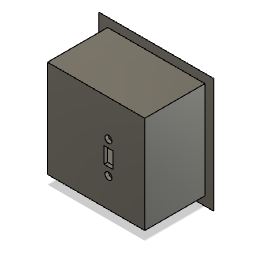
Furniture DC and USB panel v5 (Autodesk Fusion 360 design; units mm, degrees)
Autodesk Fusion 360 part; units mm, degrees
sketch "Sketch1" plane through (0, 0, 0) normal (0, 1, 0) x (1, 0, 0)
  circle A0 centre (0, 0) radius 4.075
  line L0 (26.5, -2.5) -> (17.4, -2.5)
  line L1 (17.4, -2.5) -> (17.4, 2.5)
  line L2 (17.4, 2.5) -> (26.5, 2.5)
  line L3 (26.5, 2.5) -> (26.5, -2.5)
  line L4 (26.5, -2.5) -> (17.4, 2.5) construction
  line L5 (17.4, -2.5) -> (26.5, 2.5) construction
  circle A1 centre (13, 0) radius 2
  circle A2 centre (31, 0) radius 2
  line L6 (-10, 10) -> (41, 10)
  line L7 (41, 10) -> (41, -10)
  line L8 (41, -10) -> (-10, -10)
  line L9 (-10, -10) -> (-10, 10)
  line L10 (-10, 10) -> (-12, 10)
  line L11 (-12, 10) -> (-12, -10)
  line L12 (-12, -10) -> (-10, -10)
  line L13 (-10, -10) -> (-10, 10)
  line L14 (41, 10) -> (43, 10)
  line L15 (43, 10) -> (43, -10)
  line L16 (43, -10) -> (41, -10)
  line L17 (41, -10) -> (41, 10)
  point P0 (21.95, 0)
  dimension "d1" = 8.15
  dimension "d2" = 9.1
  dimension "d3" = 5
  dimension "d4" = 4
  dimension "d5" = 4
  dimension "d6" = 18
  dimension "d7" = 9.05
  dimension "d9" = 13
  dimension "d10" = 10
  dimension "d11" = 10
  dimension "d12" = 10
  dimension "d13" = 10
  dimension "d16" = 51
  constraint coincident A0.centre origin
  constraint perpendicular L0 L1
  constraint parallel L0 L2
  constraint parallel L1 L3
  constraint horizontal L0
  constraint coincident L4 P0
  constraint coincident L5 P0
  constraint horizontal A1.centre A2.centre
  constraint horizontal P0 A2.centre
  constraint horizontal L6
  constraint vertical L7
  constraint horizontal L8
  constraint vertical L9
  constraint horizontal A0.centre A1.centre
  constraint horizontal L10
  constraint vertical L11
  constraint horizontal L12
  constraint vertical L13
  constraint horizontal L14
  constraint vertical L15
  constraint horizontal L16
  constraint vertical L17
  measures "d1" diameter of A0
  measures "d2" distance of L1.end L2.end
  measures "d3" distance of L0.end L1.end
  measures "d4" diameter of A1
  measures "d5" diameter of A2
  measures "d6" distance of A1.centre A2.centre
  measures "d7" horizontal distance of P0 A2.centre
  measures "d9" horizontal distance of A0.centre A1.centre
  measures "d10" distance of A0.centre L9
  measures "d11" distance of A2.centre L7
  measures "d12" distance of A0.centre L8
  measures "d13" distance of A0.centre L6
  measures "d16" distance of L8.end L7.end
extrude "Extrude2" add sketch "Sketch1" along normal blind 2 contours L6 L7 L8 L9 L13 L17 makes body 1
extrude "Extrude1" add sketch "Sketch1" along normal blind 2 separate body contours L6 L7 L8 L9 L13 L17 makes body 2
extrude "Extrude3" add sketch "Sketch1" along normal blind 55 contours L9 L10 L11 L12 L13 | L7 L14 L15 L16 L17 bodies 1 2
sketch "Sketch2" plane through (-10, 0, 0) normal (1, 0, 0) x (0, 0, -1)
  line L0 (-10, 2) -> (10, 2)
  line L1 (10, 2) -> (10, 55)
  line L2 (10, 55) -> (-10, 55)
  line L3 (-10, 55) -> (-10, 2)
  line L4 (-10, 55) -> (10, 55)
  line L5 (10, 55) -> (10, 53)
  line L6 (10, 53) -> (-10, 53)
  line L7 (-10, 53) -> (-10, 55)
  dimension "d21" = 2
  constraint horizontal L4
  constraint vertical L5
  constraint horizontal L6
  constraint vertical L7
  constraint coincident L1 L5.end
  constraint coincident L2.end L3.start
  measures "d21" distance of L4 L6
extrude "Extrude4" add sketch "Sketch2" along normal up to surface (51 mm away) contours L1 L2 L3 L4 L5 L6 L7 bodies 1
sketch "Sketch3" plane through (0, 0, 10) normal (0, 0, 1) x (1, 0, 0)
  line L0 (41, 53) -> (41, 2)
  line L1 (41, 2) -> (-10, 2)
  line L2 (-10, 2) -> (-10, 53)
  line L3 (-10, 53) -> (41, 53)
  line L4 (43, 55) -> (-12, 55)
  line L5 (-12, 55) -> (-12, 0)
  line L6 (-12, 0) -> (43, 0)
  line L7 (43, 0) -> (43, 55)
extrude "Extrude5" add sketch "Sketch3" along normal blind 2 contours L0 L1 L2 L3 | L4 L5 L6 L7 bodies 1
sketch "Sketch4" plane through (0, 0, -10) normal (0, 0, -1) x (-1, 0, 0)
  line L0 (12, 55) -> (-43, 55)
  line L1 (-43, 55) -> (-43, 0)
  line L2 (-43, 0) -> (12, 0)
  line L3 (12, 0) -> (12, 55)
  line L4 (-41, 53) -> (10, 53)
  line L5 (10, 53) -> (10, 2)
  line L6 (10, 2) -> (-41, 2)
  line L7 (-41, 2) -> (-41, 53)
extrude "Extrude6" add sketch "Sketch4" along normal blind 14 bodies 1
sketch "Sketch5" plane through (43, 0, 0) normal (1, 0, 0) x (0, 0, -1)
  line L0 (-12, 0) -> (24, 0)
  line L1 (24, 0) -> (24, 55)
  line L2 (24, 55) -> (-12, 55)
  line L3 (-12, 55) -> (-12, 0)
  line L4 (24, 55) -> (22, 55)
  line L5 (22, 55) -> (22, 0)
  line L6 (22, 0) -> (24, 0)
  line L7 (24, 0) -> (24, 55)
  constraint horizontal L4
  constraint vertical L5
  constraint horizontal L6
  constraint vertical L7
  constraint coincident L0 L5.end
  constraint coincident L1.end L2.start
extrude "Extrude7" add sketch "Sketch5" along normal blind 5 contours L0 L1 L2 L4 L5 L6 L7 bodies 1
sketch "Sketch6" plane through (-12, 0, 0) normal (-1, 0, 0) x (0, 0, 1)
  line L0 (-24, 0) -> (12, 0)
  line L1 (12, 0) -> (12, 55)
  line L2 (12, 55) -> (-24, 55)
  line L3 (-24, 55) -> (-24, 0)
  line L4 (-24, 55) -> (-22, 55)
  line L5 (-22, 55) -> (-22, 0)
  line L6 (-22, 0) -> (-24, 0)
  line L7 (-24, 0) -> (-24, 55)
  point P0 (-22, 0)
  constraint horizontal L4
  constraint vertical L5
  constraint horizontal L6
  constraint vertical L7
  constraint coincident P0 L5.end
  constraint coincident L2.end L3.start
extrude "Extrude8" add sketch "Sketch6" along normal blind 5 contours L0 L2 L3 L4 L5 L6 L7 bodies 1
sketch "Sketch7" plane through (0, 55, 0) normal (0, 1, 0) x (-1, 0, 0)
  line L0 (-48, -24) -> (17, -24)
  line L1 (17, -24) -> (17, -22)
  line L2 (17, -22) -> (12, -22)
  line L3 (12, -22) -> (12, 12)
  line L4 (12, 12) -> (-43, 12)
  line L5 (-43, 12) -> (-43, -22)
  line L6 (-43, -22) -> (-48, -22)
  line L7 (-48, -22) -> (-48, -24)
  line L8 (17, -22) -> (-48, -22)
  line L9 (-48, -22) -> (-48, -24)
  line L10 (-48, -24) -> (17, -24)
  line L11 (17, -24) -> (17, -22)
  constraint horizontal L8
  constraint vertical L9
  constraint horizontal L10
  constraint vertical L11
  constraint coincident L0.start L7.end
  constraint coincident L1.end L2.start
extrude "Extrude9" add sketch "Sketch7" along normal blind 5 contours L0 L1 L2 L6 L7 L8 L9 L10 L11 bodies 1
sketch "Sketch8" plane through (0, 0, 0) normal (0, -1, 0) x (1, 0, 0)
  circle A0 centre (0, 0) radius 4.075
  circle A1 centre (31, 0) radius 2
  line L0 (26.5, -2.5) -> (17.4, -2.5)
  line L1 (17.4, -2.5) -> (17.4, 2.5)
  line L2 (17.4, 2.5) -> (26.5, 2.5)
  line L3 (26.5, 2.5) -> (26.5, -2.5)
  circle A2 centre (13, 0) radius 2
  line L4 (-12, 12) -> (-12, -22)
  line L5 (-12, -22) -> (-17, -22)
  line L6 (-17, -22) -> (-17, -24)
  line L7 (-17, -24) -> (48, -24)
  line L8 (48, -24) -> (48, -22)
  line L9 (48, -22) -> (43, -22)
  line L10 (43, -22) -> (43, 12)
  line L11 (43, 12) -> (-12, 12)
  line L12 (-17, -24) -> (48, -24)
  line L13 (48, -24) -> (48, -22)
  line L14 (48, -22) -> (-17, -22)
  line L15 (-17, -22) -> (-17, -24)
  constraint horizontal L12
  constraint vertical L13
  constraint horizontal L14
  constraint vertical L15
  constraint coincident L8.end L9.start
  constraint coincident L6.end L7.start
extrude "Extrude10" add sketch "Sketch8" along normal blind 5 contours L5 L6 L7 L8 L9 L12 L13 L14 L15 bodies 1
chamfer "Chamfer1" distance 2 angle 45 4 edges at (-17, 27.5, -24) (15.5, 60, -24) (48, 27.5, -24) (15.5, -5, -24) on bodies 1
sketch "Sketch9" plane through (0, 0, 0) normal (0, 1, 0) x (-1, 0, 0)
sketch "Sketch10" plane through (0, 0, 12) normal (0, 0, 1) x (1, 0, 0)
  line L0 (43, 0) -> (43, 55)
  line L1 (43, 55) -> (-12, 55)
  line L2 (-12, 55) -> (-12, 0)
  line L3 (-12, 0) -> (43, 0)
  line L4 (19.95, 20.95) -> (19.95, 30.05)
  line L5 (19.95, 30.05) -> (24.95, 30.05)
  line L6 (24.95, 30.05) -> (24.95, 20.95)
  line L7 (24.95, 20.95) -> (19.95, 20.95)
  circle A0 centre (22.45, 16.45) radius 2
  circle A1 centre (22.45, 34.45) radius 2
  dimension "d37" = 9.1
  dimension "d38" = 5
  dimension "d39" = 4
  dimension "d40" = 4
  dimension "d41" = 18
  constraint perpendicular L4 L5
  constraint parallel L4 L6
  constraint parallel L5 L7
  measures "d37" distance of L5.end L6.end
  measures "d38" distance of L4.end L5.end
  measures "d39" diameter of A1
  measures "d40" diameter of A0
  measures "d41" distance of A0.centre A1.centre
extrude "Extrude11" cut sketch "Sketch10" against normal blind 2 contours L4 L5 L6 L7 | A0 | A1 bodies 1
extrude "Extrude12" add sketch "Sketch1" along normal blind 2 contours L0 L1 L2 L3 | A1 | A2 bodies 1
